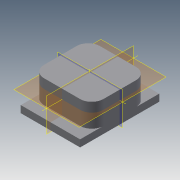
# Autodesk Inventor part: HbBatteryLockKnob01
Saved by Autodesk Inventor 2015 SP1 (Build 190203100, 203)
## iProperties
Created: 2015-03-05
Part Number: HbBatteryLockKnob01
Material: 一般
Document SubType Name: Modeling
Designer: Yamaura
Density: 1 g/cm^3
Appearance: 既定
Author: Yamaura
Autodesk Inventor part; units mm, degrees
sketch "スケッチ1" plane through (0, 0, 0) normal (0, 0, 1) x (1, 0, 0)
  line L0 (-5.1, 4.8) -> (5.1, 4.8)
  line L1 (5.1, 4.8) -> (5.1, -4.8)
  line L2 (5.1, -4.8) -> (-5.1, -4.8)
  line L3 (-5.1, -4.8) -> (-5.1, 4.8)
  point P0 (0, 0)
  dimension "d0" = 4.8
  dimension "d1" = 4.8
  dimension "d2" = 5.1
  dimension "d3" = 5.1
  constraints: 8 end point, 2 parallel, 1 horizontal, 1 perpendicular
  measures "d0" distance from line of L0 point (0, 0)
  measures "d1" distance from line of L2 point (0, 0)
  measures "d2" distance from line of L1 point (0, 0)
  measures "d3" distance from line of L3 point (0, 0)
extrude "押し出し1" add sketch "スケッチ1" along normal blind 1.6 and the other way blind 3.6
sketch "スケッチ2" plane through (0, 0, -3.6) normal (0, 0, -1) x (-1, 0, 0)
  line L0 (5.1, 4.8) -> (-5.1, 4.8) projected
  line L1 (-5.1, 4.8) -> (-5.1, -4.8) projected
  line L2 (-5.1, -4.8) -> (5.1, -4.8) projected
  line L3 (5.1, -4.8) -> (5.1, 4.8) projected
  line L4 (5.1, -6.8) -> (-5.1, -6.8)
  line L5 (-5.1, -6.8) -> (-5.1, 6.8)
  line L6 (-5.1, 6.8) -> (5.1, 6.8)
  line L7 (5.1, 6.8) -> (5.1, -6.8)
  line L8 (0, -9.52) -> (0, 9.52) projected
  point P0 (0, 0)
  dimension "d8" = 2
  dimension "d24" = 5.1
  dimension "d30" = 5.1
  constraints: 8 end point, 1 perpendicular
  measures "d8" distance between parallel lines of L2 L4
  measures "d24" distance between parallel lines of L8 L7
  measures "d30" distance from line of L5 point (0, 0)
extrude "押し出し2" add sketch "スケッチ2" against normal blind 1.2 contours L0 L8 L6 L7 | L0 L5 L6 L8 | L7 L4 L8 L2 | L8 L4 L5 L2
sketch "スケッチ3" plane through (0, 0, 0) normal (0, 0, 1) x (1, 0, 0)
  line L0 (5.1, 4.8) -> (-5.1, 4.8) projected
  line L1 (-5.1, 4.8) -> (-5.1, -4.8) projected
  line L2 (-5.1, -4.8) -> (5.1, -4.8) projected
  line L3 (5.1, -4.8) -> (5.1, 4.8) projected
  circle A0 centre (0, 0) radius 3.25
  dimension "d28" = 6.5
  constraints: 1 centre point, 1 coincident
  measures "d28" diameter of A0
extrude "押し出し3" cut sketch "スケッチ3" against normal through all contours A0
fillet "フィレット2" radius 2 4 edges at (5.1, -4.8, -0.4) (5.1, 4.8, -0.4) (-5.1, 4.8, -0.4) (-5.1, -4.8, -0.4)
